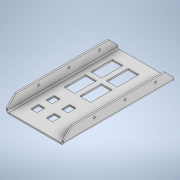
# Autodesk Inventor part: sheetmetalface
Saved by Autodesk Inventor 2020.2 (Build 242310000, 310)
## iProperties
Created: 2020-02-05
Part Number: sheetmetalface
Material: Generic
Document SubType Name: Sheet Metal
Designer: ColinP
Density: 1 g/cm^3
Sheet Metal Rule: Default
Appearance: Default
Flat Pattern Width: 16.2921 cm
Flat Pattern Length: 22.86 cm
Flat Pattern Area: 372.437 cm^2
Sheet Metal Width: 6.414 in
Sheet Metal Length: 9.000 in
Sheet Metal Area: 57.728 in^2
Author: ColinP
Autodesk Inventor part; units mm, degrees
ref_plane "YZ Plane" through (0, 0, 0) normal (1, 0, 0) x (0, 1, 0)
ref_plane "XZ Plane" through (0, 0, 0) normal (0, 1, 0) x (-1, 0, 0)
ref_plane "XY Plane" through (0, 0, 0) normal (0, 0, 1) x (1, 0, 0)
sketch "Sketch1" plane through (0, 0, 0) normal (0, 1, 0) x (-1, 0, 0)
  line L0 (0, 0) -> (127, 0)
  line L1 (127, 0) -> (127, 228.6)
  line L2 (127, 228.6) -> (0, 228.6)
  line L3 (0, 228.6) -> (0, 0)
  dimension "d0" = 127
  dimension "d1" = 228.6
  measures "d0" distance of L2.end L1.end
  measures "d1" distance of L1.end L0.end
extrude "Plate1" add sketch "Sketch1" along normal blind 3.048
sketch "Sketch2" plane through (0, 3.048, 0) normal (0, 1, 0) x (1, 0, 0)
  line L0 (0, 0) -> (-50.8, 0)
  line L1 (0, 0) -> (-127, 0) projected
  line L2 (-50.8, 0) -> (-50.8, -25.4)
  line L3 (-50.8, -25.4) -> (-73.406, -25.4)
  line L4 (-73.406, -25.4) -> (-73.406, -70.612)
  line L5 (-73.406, -70.612) -> (-50.8, -70.612)
  line L6 (-50.8, -70.612) -> (-50.8, -25.4)
  line L7 (-73.406, -25.4) -> (-83.406, -25.4)
  line L8 (-83.406, -25.4) -> (-106.012, -25.4)
  line L9 (-106.012, -25.4) -> (-106.012, -70.612)
  line L10 (-106.012, -70.612) -> (-83.406, -70.612)
  line L11 (-83.406, -70.612) -> (-83.406, -25.4)
  line L12 (-83.406, -70.612) -> (-83.406, -80.612)
  line L13 (-83.406, -80.612) -> (-106.012, -80.612)
  line L14 (-106.012, -80.612) -> (-106.012, -125.824)
  line L15 (-106.012, -125.824) -> (-83.406, -125.824)
  line L16 (-83.406, -125.824) -> (-83.406, -80.612)
  line L17 (-73.406, -80.612) -> (-50.8, -80.612)
  line L18 (-50.8, -125.824) -> (-73.406, -125.824)
  line L19 (-73.406, -80.612) -> (-73.406, -125.824)
  line L20 (-50.8, -125.824) -> (-50.8, -80.612)
  point P0 (0, -228.6)
  dimension "d3" = 50.8
  dimension "d4" = 25.4
  dimension "d5" = 22.606
  dimension "d6" = 45.212
  dimension "d7" = 10
  dimension "d8" = 22.606
  dimension "d9" = 10
  dimension "d10" = 45.212
  constraints: 40 end point, 18 point on line, 10 perpendicular, 1 parallel, 1 vertical
  measures "d3" distance of L0.start L0.end
  measures "d4" distance of L0.end L2.end
  measures "d5" distance of L2.end L3.end
  measures "d6" distance of L3.end L4.end
  measures "d7" distance of L3.end L7.end
  measures "d8" distance of L7.end L8.end
  measures "d9" distance of L10.end L12.end
  measures "d10" distance of L13.end L14.end
extrude "Cut1" cut sketch "Sketch2" against normal blind 3.048
sketch "Sketch3" plane through (0, 3.048, 0) normal (0, 1, 0) x (1, 0, 0)
  line L0 (-50.8, -125.824) -> (-73.406, -125.824) projected
  line L1 (-62.103, -125.824) -> (-62.103, -151.224)
  line L2 (0, -228.6) -> (-127, -228.6) projected
  line L3 (-62.103, -151.224) -> (-68.58, -151.224)
  line L4 (-68.58, -151.224) -> (-55.626, -151.224)
  line L5 (-68.58, -151.224) -> (-68.58, -167.988)
  line L6 (-68.58, -167.988) -> (-55.626, -167.988)
  line L7 (-55.626, -167.988) -> (-55.626, -151.224)
  line L8 (-83.406, -125.824) -> (-106.012, -125.824) projected
  line L9 (-94.709, -125.824) -> (-94.709, -151.224)
  line L10 (-94.709, -151.224) -> (-101.186, -151.224)
  line L11 (-101.186, -151.224) -> (-88.232, -151.224)
  line L12 (-88.232, -151.224) -> (-88.232, -167.988)
  line L13 (-88.232, -167.988) -> (-101.186, -167.988)
  line L14 (-101.186, -167.988) -> (-101.186, -151.224)
  line L15 (-94.709, -167.988) -> (-94.709, -183.228)
  line L16 (-94.709, -183.228) -> (-101.186, -183.228)
  line L17 (-101.186, -183.228) -> (-101.186, -199.992)
  line L18 (-101.186, -199.992) -> (-88.232, -199.992)
  line L19 (-88.232, -199.992) -> (-88.232, -183.228)
  line L20 (-88.232, -183.228) -> (-94.709, -183.228)
  line L21 (-68.58, -167.988) -> (-68.58, -183.228)
  line L22 (-68.58, -183.228) -> (-55.626, -183.228)
  line L23 (-55.626, -183.228) -> (-55.626, -199.992)
  line L24 (-55.626, -199.992) -> (-68.58, -199.992)
  line L25 (-68.58, -199.992) -> (-68.58, -183.228)
  point P0 (0, 0)
  dimension "d25" = 25.4
  dimension "d26" = 6.477
  dimension "d27" = 12.954
  dimension "d28" = 16.764
  dimension "d29" = 6.477
  dimension "d30" = 12.954
  dimension "d31" = 15.24
  dimension "d32" = 16.764
  constraints: 46 end point, 13 perpendicular, 5 point on line, 4 vertical, 3 midpoint, 2 parallel, 1 horizontal
  measures "d25" distance of L1.start L1.end
  measures "d26" distance of L1.end L3.end
  measures "d27" distance of L3.end L4.end
  measures "d28" distance of L3.end L5.end
  measures "d29" distance of L9.end L10.end
  measures "d30" distance of L10.end L11.end
  measures "d31" distance of L15.start L15.end
  measures "d32" distance of L16.end L17.end
extrude "Cut2" cut sketch "Sketch3" against normal blind 3.048
sketch "Sketch4" plane through (0, 3.048, 0) normal (0, 1, 0) x (1, 0, 0)
  line L0 (-127, 0) -> (-127, -228.6)
  line L1 (-127, -228.6) -> (-144.9605, -210.6395)
  line L2 (-127, -228.6) -> (-101.6, -228.6) construction
  line L3 (-127, 0) -> (-144.9605, -17.9605)
  line L4 (-144.9605, -17.9605) -> (-144.9605, -210.6395)
  point P0 (0, 0)
  dimension "d35" = 25.4
  dimension "d36" = 135
  dimension "d37" = 25.4
  measures "d35" distance of L0.end L1.end
  measures "d36" angle of L2 L1
  measures "d37" distance of L0.start L3.end
sheet face with bend "Face2" sketch "Sketch4" thickness 3.048 toward (0, -1, 0) bend radius 3.048
bend "Bend1"
sketch "Sketch8" plane through (0, 3.048, 0) normal (0, 1, 0) x (1, 0, 0)
  line L0 (0, 0) -> (17.9605, -17.9605)
  line L1 (0, 0) -> (25.4, 0) construction
  line L2 (0, 0) -> (0, -228.6)
  line L3 (0, -228.6) -> (17.9605, -210.6395)
  line L4 (0, -228.6) -> (25.4, -228.6) construction
  line L5 (17.9605, -210.6395) -> (17.9605, -17.9605)
  dimension "d49" = 25.4
  dimension "d50" = 45
  dimension "d51" = 25.4
  dimension "d52" = 45
  measures "d49" distance of L0.start L0.end
  measures "d50" angle of L0 L1
  measures "d51" distance of L2.end L3.end
  measures "d52" angle of L4 L3
sheet face with bend "Face3" sketch "Sketch8" thickness 3.048 toward (0, -1, 0) bend radius 3.048
bend "Bend2"
sketch "Sketch10" plane through (0, 3.048, 0) normal (0, -1, 0) x (1, 0, 0)
  line L0 (0, 0) -> (-127, 0) projected
  line L1 (-127, 0) -> (-120.65, 0)
  line L2 (-120.65, 0) -> (-120.65, 228.6)
  line L3 (0, 228.6) -> (-127, 228.6) projected
  line L4 (-120.65, 228.6) -> (-120.65, 0)
  dimension "d65" = 6.35
  constraints: 6 end point, 2 point on line, 1 perpendicular, 1 vertical
  measures "d65" distance of L0.end L1.end
fold "Fold5" angle 90 bend radius 3.048 thickness 3.048 k factor 0.44 line from (-120.65, 3.048, 0) to (-120.65, 3.048, 228.6) line at bend centre moving side (1, 0, 0) folds toward (0, 1, 0)
sketch "Sketch12" plane through (-121.0492, 141.2593, 17.9605) normal (-1, 0, 0) x (0, 0, 1)
  line L0 (210.6395, -17.9605) -> (210.6395, -135.1633) projected
  line L1 (210.6395, -17.9605) -> (210.6395, -24.3105)
  line L2 (210.6395, -24.3105) -> (-17.9605, -24.3105)
  line L3 (-17.9605, -17.9605) -> (-17.9605, -135.1633) projected
  point P0 (-17.9605, -141.2593)
  dimension "d84" = 6.35
  constraints: 4 end point, 2 point on line, 1 perpendicular
  measures "d84" distance of L0.start L1.end
fold "Fold6" angle 90 bend radius 3.048 thickness 3.048 k factor 0.44 line from (-121.0492, 116.9488, 228.6) to (-121.0492, 116.9488, 0) line at bend centre moving side (0, -1, 0) folds toward (-1, 0, 0)
sketch "Sketch13" plane through (-118.0012, 141.2593, 17.9605) normal (-1, 0, 0) x (0, 0, 1)
  line L0 (210.6395, -17.9605) -> (210.6395, -20.8633) projected
  line L1 (210.6395, -17.9605) -> (210.6395, -7.8005)
  line L2 (210.6395, -7.8005) -> (147.1395, -7.8005)
  line L3 (147.1395, -7.8005) -> (83.6395, -7.8005)
  line L4 (83.6395, -7.8005) -> (20.1395, -7.8005)
  point P0 (-17.9605, -141.2593)
  dimension "d91" = 10.16
  dimension "d92" = 63.5
  dimension "d93" = 63.5
  dimension "d94" = 63.5
  constraints: 8 end point, 2 point on line, 1 perpendicular, 1 vertical
  measures "d91" distance of L0.start L1.end
  measures "d92" distance of L1.end L2.end
  measures "d93" distance of L2.end L3.end
  measures "d94" distance of L3.end L4.end
hole "Hole1" at (-118.0012, 133.4588, 165.1) at (-118.0012, 133.4588, 101.6) at (-118.0012, 133.4588, 38.1) direction (-1, 0, 0) diameter 4.4958 end through all clearance for "Flat Head Machine Screw (82)" size "#8" standard "Ansi Unified Screw Threads"
equation "\"d23\" = Thickness"
equation "\"d33\" = Thickness"
equation "\"d2\" = Thickness"
equation "\"d78\" = BendReliefWidth"
equation "\"d79\" = BendReliefDepth"
equation "\"d80\" = MinimumRemnant"
equation "\"d81\" = TransitionRadius"
equation "\"d83\" = BendRadius"
equation "\"d85\" = BendReliefWidth"
equation "\"d86\" = BendReliefDepth"
equation "\"d87\" = MinimumRemnant"
equation "\"d88\" = TransitionRadius"
equation "\"d90\" = BendRadius"
equation "\"d100\" = Thickness"
equation "\"d38\" = BendRadius"
equation "\"d39\" = BendReliefWidth"
equation "\"d41\" = MinimumRemnant"
equation "\"d40\" = BendReliefDepth"
equation "\"d42\" = TransitionRadius"
equation "\"d53\" = BendRadius"
equation "\"d54\" = BendReliefWidth"
equation "\"d56\" = MinimumRemnant"
equation "\"d55\" = BendReliefDepth"
equation "\"d57\" = TransitionRadius"
equation "\"BendRadius\" = Thickness"
equation "\"BendReliefWidth\" = Thickness"
equation "\"BendReliefDepth\" = 0.5 * Thickness"
equation "\"CornerReliefSize\" = 4 * Thickness"
equation "\"MinimumRemnant\" = 2 * Thickness"
equation "\"TransitionRadius\" = BendRadius"
equation "\"JacobiRadiusSize\" = BendRadius"
equation "\"GapSize\" = Thickness"
equation "\"Thickness\" = 3.048"
body "Solid1"
